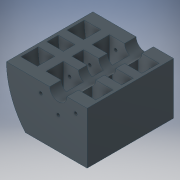
# Autodesk Inventor part: SJ005
Saved by Autodesk Inventor 2017 SP1 (Build 210196100, 196)
## iProperties
Created: 2017-06-04
Part Number: SJ005
Material: ABS Plastic
Document SubType Name: Modeling
Designer: Zach
Density: 1.06 g/cm^3
Appearance: CR Dark Blue
Author: Zach
Autodesk Inventor part; units mm, degrees
ref_plane "YZ Plane" through (0, 0, 0) normal (1, 0, 0) x (0, 1, 0)
ref_plane "XZ Plane" through (0, 0, 0) normal (0, 1, 0) x (-1, 0, 0)
ref_plane "XY Plane" through (0, 0, 0) normal (0, 0, 1) x (1, 0, 0)
sketch "Sketch1" plane through (0, 0, 0) normal (0, 0, 1) x (1, 0, 0)
  circle A0 centre (0, 90) radius 140 construction
  line L0 (0, -50) -> (0, 0) construction
  line L1 (0, 0) -> (-107.2381, 0) construction
  arc A1 (-140, 90) -> (-107.2381, 0) centre (0, 90) ccw
  line L2 (-140, 90) -> (0, 90)
  line L3 (0, 90) -> (0, 0)
  line L4 (-107.2381, 0) -> (0, 0)
  dimension "d0" = 280
  dimension "d1" = 50
  constraints: 10 end point, 5 point on circle, 2 centre point, 2 perpendicular, 1 coincident, 1 collinear, 1 concentric, 1 horizontal, 1 vertical
  measures "d0" diameter of A0
  measures "d1" distance of L0.start L0.end
extrude "Extrusion1" add sketch "Sketch1" along normal blind 150
sketch "Sketch6" plane through (-140, 90, 0) normal (0, 1, 0) x (1, 0, 0)
  line L0 (0, 0) -> (0, -150) projected
  line L1 (0, 0) -> (140, 0)
  line L2 (140, 0) -> (140, -150)
  line L3 (140, -150) -> (0, -150)
  line L4 (0, -150) -> (0, 0)
  line L5 (5, -145) -> (135, -145)
  line L6 (135, -145) -> (135, -5)
  line L7 (135, -5) -> (5, -5)
  line L8 (5, -5) -> (5, -145)
  dimension "d25" = 5
  constraints: 16 end point, 4 parallel, 2 perpendicular, 1 horizontal, 3 other
  measures "d25" distance between parallel lines of L3 L5
extrude "Extrusion5" cut sketch "Sketch6" against normal blind 85 contours L8 L7 L6 L5
sketch "Sketch7" plane through (-107.2381, 0, 0) normal (0, -1, 0) x (1, 0, 0)
  circle A0 centre (35, 115) radius 2.5
  circle A1 centre (85, 115) radius 2.5
  line L0 (0, 150) -> (107.2381, 150) projected
  line L1 (0, 0) -> (0, 150) projected
  circle A2 centre (35, 35) radius 2.5
  circle A3 centre (85, 35) radius 2.5
  line L2 (107.2381, 0) -> (107.2381, 150) projected
  dimension "d28" = 5
  dimension "d29" = 5
  dimension "d30" = 35
  dimension "d31" = 50
  dimension "d33" = 5
  dimension "d34" = 5
  dimension "d35" = 80
  dimension "d39" = 35
  constraints: 4 centre point, 2 horizontal alignment, 2 vertical alignment
  measures "d28" diameter of A0
  measures "d29" diameter of A1
  measures "d30" distance from line of L0 A0.centre
  measures "d31" distance of A1.centre A0.centre
  measures "d33" diameter of A2
  measures "d34" diameter of A3
  measures "d35" distance of A2.centre A0.centre
  measures "d39" distance from line of L1 A0.centre
extrude "Extrusion6" cut sketch "Sketch7" against normal through all
sketch "Sketch8" plane through (0, 0, 150) normal (0, 0, 1) x (1, 0, 0)
  line L0 (0, 90) -> (-140, 90) projected
  arc A0 (-140, 90) -> (-107.2381, 0) centre (0, 90) ccw projected
  arc A1 (-140, 90) -> (-107.2381, 0) centre (0, 90) ccw
  line L1 (-107.2381, 0) -> (-102.2381, 0)
  line L2 (-107.2381, 0) -> (0, 0) projected
  line L3 (-140, 90) -> (-135, 90)
  arc A2 (-135, 90) -> (-102.2381, 0) centre (5, 90) ccw
  dimension "d40" = 5
  dimension "d41" = 5
  dimension "d42" = 140
  constraints: 4 end point, 4 point on circle, 2 centre point, 2 point on line
  measures "d40" distance of L1.start L1.end
  measures "d41" distance of L0.end L3.end
  measures "d42" radius of A2
extrude "Extrusion7" add sketch "Sketch8" against normal blind 150
sketch "Sketch11" plane through (-140, 5, 0) normal (0, 1, 0) x (1, 0, 0)
  line L0 (135, -5) -> (135, -145) projected
  line L1 (135, -50) -> (5, -50)
  line L2 (5, -50) -> (5, -65)
  line L3 (5, -65) -> (135, -65)
  line L4 (135, -65) -> (135, -50)
  line L5 (135, -85) -> (5, -85)
  line L6 (5, -85) -> (5, -100)
  line L7 (5, -100) -> (135, -100)
  line L8 (135, -100) -> (135, -85)
  line L9 (32.7619, 0) -> (32.7619, -150)
  line L10 (135, -130) -> (5, -130)
  line L11 (5, -130) -> (5, -145)
  line L12 (5, -145) -> (135, -145)
  line L13 (135, -145) -> (135, -130)
  line L14 (135, -20) -> (5, -20)
  line L15 (5, -20) -> (5, -5)
  line L16 (5, -5) -> (135, -5)
  line L17 (135, -5) -> (135, -20)
  line L18 (5, -5) -> (135, -5)
  line L19 (5, -145) -> (5, -5) projected
  line L20 (135, -145) -> (5, -145) projected
  line L21 (135, -5) -> (135, -20)
  point P0 (140, 0)
  point P1 (70, -145)
  point P2 (70, -5)
  point P3 (5, -12.5)
  point P4 (5, -57.5)
  dimension "d54" = 15
  dimension "d55" = 15
  dimension "d56" = 15
  dimension "d57" = 15
  dimension "d58" = 30
  dimension "d59" = 30
  dimension "d66" = 5
  constraints: 38 end point, 8 parallel, 8 point on line, 6 midpoint, 4 horizontal, 4 perpendicular, 1 collinear
  measures "d54" distance of L2.end L1.end
  measures "d55" distance of L6.end L5.end
  measures "d56" distance between parallel lines of L12 L10
  measures "d57" distance between parallel lines of L16 L14
  measures "d58" distance between parallel lines of L14 L1
  measures "d59" distance between parallel lines of L10 L7
  measures "d66" distance from line of point (140, 0) L18
extrude "Extrusion10" add sketch "Sketch11" along normal blind 85 contours L0 L14 L9 L16 | L9 L14 L15 L16 | L0 L3 L9 L1 | L9 L3 L2 L1 | L0 L7 L9 L5 | L9 L7 L6 L5 | L0 L12 L9 L10 | L9 L12 L11 L10
sketch "Sketch12" plane through (-140, 5, 0) normal (0, 1, 0) x (1, 0, 0)
  line L0 (32.7619, 0) -> (140, 0) projected
  line L1 (32.7619, -150) -> (140, -150) projected
  line L2 (83.5578, 0) -> (98.5578, 0)
  line L3 (98.5578, 0) -> (98.5578, -150)
  line L4 (98.5578, -150) -> (83.5578, -150)
  line L5 (83.5578, -150) -> (83.5578, 0)
  line L6 (33.757, 0) -> (48.757, 0)
  line L7 (48.757, 0) -> (48.757, -150)
  line L8 (48.757, -150) -> (33.757, -150)
  line L9 (33.757, -150) -> (33.757, 0)
  dimension "d62" = 15
  dimension "d63" = 15
  constraints: 16 end point, 4 parallel, 4 point on line, 2 horizontal, 2 perpendicular
  measures "d62" distance of L3.end L4.end
  measures "d63" distance of L7.end L8.end
extrude "Extrusion11" add sketch "Sketch12" along normal blind 85 contours L0 L7 L1 L9 | L0 L3 L1 L5
sketch "Sketch9" plane through (0, 0, 150) normal (0, 0, 1) x (1, 0, 0)
  circle A0 centre (-50, 90) radius 15
  point P0 (0, 0)
  point P1 (0, 90)
  dimension "d45" = 30
  dimension "d46" = 50
  constraints: 1 centre point, 1 horizontal alignment
  measures "d45" diameter of A0
  measures "d46" horizontal distance of A0.centre point (0, 0)
extrude "Extrusion8" cut sketch "Sketch9" against normal through all
sketch "Sketch13" plane through (0, 0, 0) normal (0, 0, -1) x (-1, 0, 0)
  arc A0 (107.2381, 0) -> (140, 90) centre (0, 90) ccw
  line L0 (140, 90) -> (140, 90)
  arc A1 (107.2381, 0) -> (140, 90) centre (0, 90) ccw projected
  line L1 (140, 90) -> (140, 90)
  line L2 (65, 90) -> (140, 90) projected
  line L3 (140, 90) -> (140, 0)
  line L4 (140, 0) -> (107.2381, 0)
  point P0 (0, 0)
  dimension "d67" = 140
  constraints: 8 end point, 2 perpendicular, 2 point on circle, 2 vertical, 1 centre point, 1 tangent
  measures "d67" radius of A0
extrude "Extrusion12" cut sketch "Sketch13" against normal through all
sketch "Sketch14" plane through (0, 0, 150) normal (0, 0, 1) x (1, 0, 0)
  line L0 (-107.2381, 0) -> (0, 0) construction
  line L1 (-50, 0) -> (-50, 196.0469) construction
  line L2 (0, 90) -> (-93.0222, 90) construction
  line L3 (-50, 90) -> (28.9192, 90) construction
  circle A0 centre (-50, 125) radius 2.5
  circle A1 centre (-50, 90) radius 35 construction
  circle A2 centre (-80.3109, 107.5) radius 2.5
  circle A3 centre (-80.3109, 72.5) radius 2.5
  circle A4 centre (-50, 55) radius 2.5
  circle A5 centre (-19.6891, 72.5) radius 2.5
  circle A6 centre (-19.6891, 107.5) radius 2.5
  dimension "d74" = 70
  dimension "d70" = 50
  dimension "d72" = 5
  dimension "d77" = 360
  constraints: 6 centre point, 6 end point, 4 point on line, 2 horizontal, 1 coincident, 1 perpendicular, 1 vertical alignment, 15 other
  measures "d70" distance from line of L0.end L1
  measures "d72" diameter of A0
extrude "Extrusion13" cut sketch "Sketch14" against normal through all contours A3 | A4 | A5
body "Solid1"
